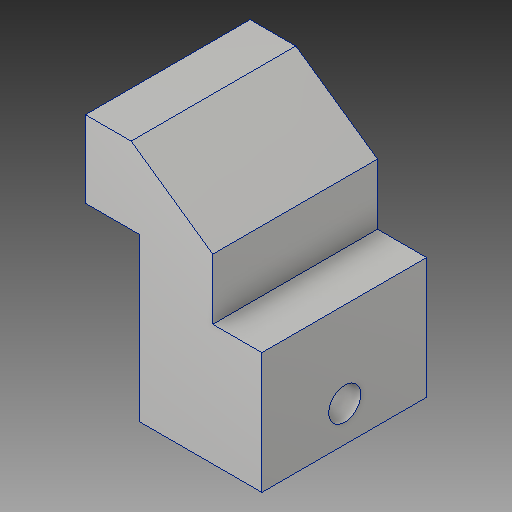
# Autodesk Inventor part: 小虎鉗-右側
Saved by Autodesk Inventor 2017 (Build 210142000, 142)
## iProperties
Part Number: 小虎鉗-右側
Material: 鋁合金 6061
Document SubType Name: Modeling
Designer: user
Density: 2.7 g/cm^3
Appearance: 鋁 - 平面
Author: user
Autodesk Inventor part; units mm, degrees
ref_plane "YZ Plane" through (0, 0, 0) normal (1, 0, 0) x (0, 1, 0)
ref_plane "XZ Plane" through (0, 0, 0) normal (0, 1, 0) x (-1, 0, 0)
ref_plane "XY Plane" through (0, 0, 0) normal (0, 0, 1) x (1, 0, 0)
sketch "草圖1" plane through (0, 0, 0) normal (0, 0, 1) x (1, 0, 0)
  line L0 (20.5635, 0) -> (58.6435, 0)
  line L1 (58.6435, 0) -> (58.6435, 37.62)
  line L2 (58.6435, 37.62) -> (43.3835, 37.62)
  line L3 (43.3835, 37.62) -> (43.3835, 56.4986)
  line L4 (43.3835, 56.4986) -> (17.9968, 74.2368)
  line L5 (17.9968, 74.2368) -> (3.7768, 74.2368)
  line L6 (3.7768, 74.2368) -> (3.7768, 50.4)
  line L7 (3.7768, 50.4) -> (20.5635, 50.4)
  line L8 (20.5635, 50.4) -> (20.5635, 0)
  point P0 (0, 0)
  dimension "d0" = 38.08
  dimension "d1" = 37.62
  dimension "d2" = 15.26
  dimension "d3" = 50.4
  dimension "d4" = 14.22
  constraints: 18 end point, 6 perpendicular, 1 horizontal, 1 parallel
  measures "d0" distance of L0.start L0.end
  measures "d1" distance of L0.end L1.end
  measures "d2" distance of L1.end L2.end
  measures "d3" distance between parallel lines of L0 L7
  measures "d4" distance of L4.end L5.end
extrude "擠出1" add sketch "草圖1" along normal blind 51.2
sketch "草圖2" plane through (58.6435, 0, 0) normal (1, 0, 0) x (0, 0, -1)
  circle A0 centre (-25.46, 11) radius 5
  line L0 (0, 37.62) -> (0, 0) projected
  line L1 (0, 0) -> (-51.2, 0) projected
  dimension "d7" = 10
  dimension "d8" = 25.46
  dimension "d9" = 11
  constraints: 1 centre point
  measures "d7" diameter of A0
  measures "d8" distance from line of L0 A0.centre
  measures "d9" distance from line of A0.centre L1
extrude "擠出2" cut sketch "草圖2" against normal blind 51.2
sketch "草圖3" plane through (20.5635, 0, 0) normal (-1, 0, 0) x (0, 0, 1)
  line L0 (39.2, 0) -> (39.2, 24.4)
  line L1 (39.2, 24.4) -> (12.2, 24.4)
  line L2 (12.2, 24.4) -> (12.2, 0)
  line L3 (51.2, 50.4) -> (51.2, 0) projected
  line L4 (12.2, 0) -> (12.2, -12.2233)
  line L5 (12.2, -12.2233) -> (39.2, -4.7386)
  line L6 (39.2, -4.7386) -> (39.2, 0)
  dimension "d12" = 27
  dimension "d13" = 12
  constraints: 12 end point, 2 parallel, 1 vertical
  measures "d12" distance of L0.end L1.end
  measures "d13" distance between parallel lines of L3 L0
extrude "擠出3" cut sketch "草圖3" against normal blind 29.64
